feets_v4 (Autodesk Fusion 360 design; units mm, degrees)
Autodesk Fusion 360 part; units mm, degrees
sketch "Esquisse1" plane through (0, 0, 0) normal (0, 0, 1) x (1, 0, 0) in component "feet"
  circle A0 centre (0, 0) radius 20
  circle A1 centre (0, 0) radius 10
  dimension "d1" = 40
  dimension "d2" = 20
  constraint coincident A0.centre A1.centre
  measures "d1" diameter of A0
  measures "d2" diameter of A1
extrude "Extrusion1" add sketch "Esquisse1" along normal blind 5 makes body 1 in component "feet"
extrude "Extrusion2" add sketch "Esquisse1" along normal blind 35 contours A1 bodies 1 in component "feet"
sketch "Esquisse1 (2)" plane through (0, 0, 35) normal (0, 0, 1) x (-1, 0, 0) in component "Component"
  circle A0 centre (0, 0) radius 10
  circle A1 centre (0, 0) radius 10.1
  circle A2 centre (0, 0) radius 13.1
  circle A3 centre (0, 0) radius 20
  dimension "d7" = 0.1
  dimension "d8" = 3.1
extrude "Extrusion1'" add sketch "Esquisse1 (2)" against normal blind 5 separate body contours A3 makes body 2 in component "Component"
extrude "Extrusion2'" add sketch "Esquisse1 (2)" against normal blind 30 contours A2 bodies 2 in component "Component"
ref_plane "Plan de construction1" through (0, -13.1, 13.2652) normal (0, -1, 0) x (1, 0, 0) in component "Component"
sketch "Esquisse2" plane through (0, -13.1, 13.2652) normal (0, -1, 0) x (1, 0, 0) in component "Component"
  circle A0 centre (0, -2.2652) radius 2.5
  line L0 (-13.1, -8.2652) -> (13.1, -8.2652)
  line L1 (0, 22) -> (0, -8.2652) construction
  dimension "d20" = 5
  dimension "d21" = 6
  constraint midpoint L0 L1.end
  constraint perpendicular L0 L1
  constraint coincident A0.centre L1
  measures "d20" diameter of A0
  measures "d21" distance of A0.centre L0
sketch "Esquisse3" plane through (0, 0, 30) normal (0, 0, -1) x (1, 0, 0) in component "Component"
  circle A0 centre (0, 0) radius 13.1
  circle A1 centre (0, 0) radius 20
  line L0 (5, 27.5) -> (-5, 27.5)
  line L1 (-5, 27.5) -> (-5, -27.5)
  line L2 (-5, -27.5) -> (5, -27.5)
  line L3 (5, -27.5) -> (5, 27.5)
  line L4 (5, 27.5) -> (-5, -27.5) construction
  line L5 (-5, 27.5) -> (5, -27.5) construction
  dimension "d24" = 10
  constraint horizontal L0
  constraint perpendicular L0 L1
  constraint parallel L0 L2
  constraint parallel L1 L3
  constraint coincident L4 A0.centre
  constraint coincident L5 A0.centre
  constraint coincident A0.centre A1.centre
  measures "d24" distance of L1.end L2.end
extrude "Extrusion4" add sketch "Esquisse3" along normal up to surface (25 mm away) contours A0 A1 L1 L3 | A0 A1 L1 L3 bodies 2 in component "Component"
extrude "Extrusion3" [suppressed] in component "feet"
extrude "Extrusion3'" cut sketch "Esquisse2" along normal through all and the other way through all bodies 2 in component "Component"
component "feet" placed x (1, 0, 0) y (0, 1, 0) z (0, 0, 1) at (0, 0, 0)
component "Component" placed x (1, 0, 0) y (0, 1, 0) z (0, 0, 1) at (0, 0, 20)
equation "d8 = 3 mm + 0.1 mm"
